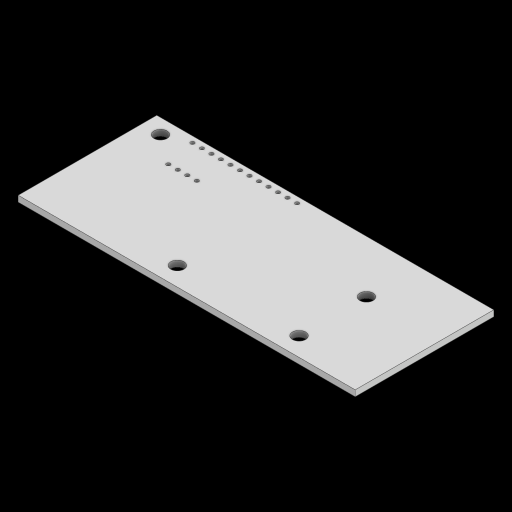
# Autodesk Inventor part: 110_PICO_Daughterboard
Saved by Autodesk Inventor 2024 (Build 280153000, 153)
## iProperties
Created: 2023-07-20
Part Number: 110_PICO_Daughterboard
Material: Generisch
Document SubType Name: Modeling
Designer: Philipp
Density: 1 g/cm^3
Appearance: Vorgabe
Author: Philipp
Autodesk Inventor part; units mm, degrees
ref_plane "YZ Plane" through (0, 0, 0) normal (1, 0, 0) x (0, 1, 0)
ref_plane "XZ Plane" through (0, 0, 0) normal (0, 1, 0) x (-1, 0, 0)
ref_plane "XY Plane" through (0, 0, 0) normal (0, 0, 1) x (1, 0, 0)
sketch "Skizze1" plane through (0, 0, 0) normal (0, 0, 1) x (1, 0, 0)
  line L0 (0, 0) -> (90, 0)
  line L1 (90, 0) -> (90, 37)
  line L2 (90, 37) -> (0, 37)
  line L3 (0, 37) -> (0, 0)
  dimension "d0" = 90
  dimension "d1" = 37
  constraints: 8 end point, 2 parallel, 1 horizontal, 1 perpendicular
  measures "d0" distance of L2.end L1.end
  measures "d1" distance of L1.end L0.end
extrude "Extrusion1" add sketch "Skizze1" against normal blind 1.6
sketch "Skizze2" plane through (0, 0, 0) normal (0, 0, 1) x (1, 0, 0)
  circle A0 centre (5, 33) radius 1.75
  circle A1 centre (37.5, 5) radius 1.75
  circle A2 centre (70, 5) radius 1.75
  circle A3 centre (70, 23) radius 1.75
  line L0 (0, 0) -> (90, 0) projected
  line L1 (0, 37) -> (0, 0) projected
  line L2 (90, 0) -> (90, 37) projected
  dimension "d4" = 3.5
  dimension "d5" = 3.5
  dimension "d6" = 3.5
  dimension "d7" = 3.5
  dimension "d8" = 33
  dimension "d9" = 5
  dimension "d10" = 37.5
  dimension "d11" = 5
  dimension "d12" = 5
  dimension "d14" = 70
  dimension "d15" = 70
  dimension "d16" = 23
  constraints: 4 centre point
  measures "d4" diameter of A0
  measures "d5" diameter of A1
  measures "d6" diameter of A2
  measures "d7" diameter of A3
  measures "d8" distance from line of L0 A0.centre
  measures "d9" distance from line of L1 A0.centre
  measures "d10" distance from line of L1 A1.centre
  measures "d11" distance from line of L0 A1.centre
  measures "d12" distance from line of L0 A2.centre
  measures "d14" distance from line of L1 A2.centre
  measures "d15" distance from line of L1 A3.centre
  measures "d16" distance from line of L0 A3.centre
extrude "Extrusion2" cut sketch "Skizze2" against normal blind 1.6
sketch "Skizze3" plane through (0, 0, 0) normal (0, 0, 1) x (1, 0, 0)
  circle A0 centre (11.152, 35.373) radius 0.5
  line L0 (0, 0) -> (90, 0) projected
  line L1 (0, 37) -> (0, 0) projected
  circle A1 centre (12.889, 27.192) radius 0.5
  dimension "d19" = 1
  dimension "d20" = 35.373
  dimension "d21" = 11.152
  dimension "d22" = 1
  dimension "d23" = 27.192
  dimension "d24" = 12.889
  constraints: 2 centre point
  measures "d19" diameter of A0
  measures "d20" distance from line of L0 A0.centre
  measures "d21" distance from line of L1 A0.centre
  measures "d22" diameter of A1
  measures "d23" distance from line of L0 A1.centre
  measures "d24" distance from line of L1 A1.centre
extrude "Extrusion3" cut sketch "Skizze3" against normal blind 1.6
pattern_linear "Rechteckige Anordnung1" count 12 spacing 2.54 along (1, 0, 0) of "Extrusion3"
sketch "Skizze4" plane through (0, 0, 0) normal (0, 0, 1) x (1, 0, 0)
  line L0 (21.549, 28.192) -> (42.329, 28.192)
  line L1 (42.329, 28.192) -> (42.329, 26.192)
  line L2 (42.329, 26.192) -> (21.549, 26.192)
  line L3 (21.549, 26.192) -> (21.549, 28.192)
  circle A0 centre (23.049, 27.192) radius 0.5 projected
  circle A1 centre (40.829, 27.192) radius 0.5 projected
  point P0 (0, 0)
  dimension "d30" = 1
  dimension "d31" = 1
  dimension "d32" = 1
  dimension "d33" = 1
  constraints: 8 end point, 2 parallel, 1 horizontal, 1 perpendicular
  measures "d30" distance edge to line of A0 L3
  measures "d31" distance edge to line of A1 L1
  measures "d32" distance from line of A0.centre L2
  measures "d33" distance from line of L0 A0.centre
extrude "Extrusion4" add sketch "Skizze4" against normal blind 1.6 contours L0 L1 L2 L3 | A0 | A1
